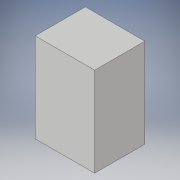
# Autodesk Inventor part: SizingCube
Saved by Autodesk Inventor 2019 (Build 230136000, 136)
## iProperties
Created: 2019-01-09
Part Number: SizingCube
Material: Generic
Document SubType Name: Modeling
Designer: james
Density: 1 g/cm^3
Appearance: Default
Author: james
Autodesk Inventor part; units mm, degrees
ref_plane "YZ Plane" through (0, 0, 0) normal (1, 0, 0) x (0, 1, 0)
ref_plane "XZ Plane" through (0, 0, 0) normal (0, 1, 0) x (-1, 0, 0)
ref_plane "XY Plane" through (0, 0, 0) normal (0, 0, 1) x (1, 0, 0)
sketch "Sketch1" plane through (0, 0, 0) normal (0, 1, 0) x (-1, 0, 0)
  line L0 (465.8955, 290.155) -> (-346.9045, 290.155)
  line L1 (-346.9045, 290.155) -> (-346.9045, -395.645)
  line L2 (-346.9045, -395.645) -> (465.8955, -395.645)
  line L3 (465.8955, -395.645) -> (465.8955, 290.155)
  point P0 (0, 0)
  dimension "d0" = 812.8
  dimension "d1" = 685.8
  constraints: 8 end point, 2 parallel, 1 horizontal, 1 perpendicular
  measures "d0" distance of L0.start L0.end
  measures "d1" distance of L0.end L1.end
extrude "Extrusion1" add sketch "Sketch1" along normal blind 1219.2
body "Solid1"
